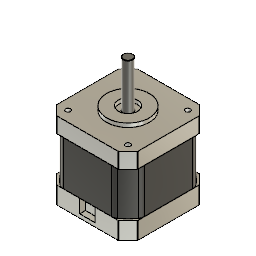
AquaMOCO-Slider-1-0-0 (Autodesk Fusion 360 archive; units mm, degrees)
design "Nema17_40mm_V2"
Autodesk Fusion 360 part; units mm, degrees
note: some values were not read from the file. Chosen so that the rebuilt part matches the saved one: how an offset face is resized.
sketch "Sketch1" plane through (0, 0, 0) normal (0, 0, 1) x (1, 0, 0) in component "Component"
  line L0 (16, 21) -> (-16, 21)
  line L1 (-21, 16) -> (-21, -16)
  line L2 (-16, -21) -> (16, -21)
  line L3 (21, -16) -> (21, 16)
  line L4 (21, 21) -> (-21, -21) construction
  line L5 (-21, 21) -> (21, -21) construction
  line L6 (-15.6506, 22.8547) -> (-16, 22.8547)
  line L7 (-21, 16) -> (-16, 21)
  line L8 (21, 16) -> (16, 21)
  line L9 (-16, -21) -> (-21, -16)
  line L10 (16, -21) -> (21, -16)
  circle A0 centre (-15.5, 15.5) radius 1.5
  circle A1 centre (15.5, 15.5) radius 1.5
  circle A2 centre (15.5, -15.5) radius 1.5
  circle A3 centre (-15.5, -15.5) radius 1.5
  circle A4 centre (0, 0) radius 11
  circle A5 centre (0, 0) radius 5
  circle A6 centre (0, 0) radius 2.5
  line L11 (-15.5, 15.5) -> (24, 15.5) construction
  line L12 (-15.5, -15.5) -> (24, -15.5) construction
  line L13 (15.5, 29) -> (15.5, -23) construction
  dimension "d3" = 3
  dimension "d4" = 15.5
  dimension "d5" = 15.5
  dimension "d6" = 5
  dimension "d58" = 15.5
  measures "d3" diameter of A0
  measures "d4" distance of A4.centre A0.centre
  measures "d5" distance of A4.centre A0.centre
  measures "d6" diameter of A6
  measures "d58" distance of A4.centre L13
extrude "Extrude1" add sketch "Sketch1" along normal blind 2 contours A4 makes body 1 in component "Component"
extrude "Extrude2" add sketch "Sketch1" along normal blind 24 separate body contours A6 makes body 2 in component "Component"
extrude "Extrude3" add sketch "Sketch1" against normal blind 1 separate body contours A5 makes body 3 in component "Component"
extrude "Extrude4" add sketch "Sketch1" against normal blind 8 contours L0 L1 L2 L3 L7 L8 L9 L10 | A4 bodies 1 3 in component "Component"
sketch "Sketch2" plane through (0, 0, -8) normal (0, 0, -1) x (1, 0, 0) in component "Component"
  circle A0 centre (15.5, 15.5) radius 1.5
  circle A1 centre (15.5, -15.5) radius 1.5
  circle A2 centre (0, 0) radius 5
  circle A3 centre (-15.5, 15.5) radius 1.5
  circle A4 centre (-15.5, -15.5) radius 1.5
  line L0 (16, 21) -> (-16, 21)
  line L1 (-16, 21) -> (-21, 16)
  line L2 (-21, 16) -> (-21, -16)
  line L3 (-21, -16) -> (-16, -21)
  line L4 (-16, -21) -> (16, -21)
  line L5 (16, -21) -> (21, -16)
  line L6 (21, -16) -> (21, 16)
  line L7 (21, 16) -> (16, 21)
  line L8 (12.4984, 21) -> (-12.4984, 21)
  line L9 (-21, 12.4984) -> (-21, -12.4984)
  line L10 (-12.4984, -21) -> (12.4984, -21)
  line L11 (21, -12.4984) -> (21, 12.4984)
  line L12 (21, 21) -> (-21, -21) construction
  line L13 (-21, 21) -> (21, -21) construction
  arc A5 (-14.8678, 20.2227) -> (-20.2227, 14.8678) centre (0, 0) ccw
  arc A6 (20.2227, 14.8678) -> (14.8678, 20.2227) centre (0, 0) ccw
  arc A7 (-20.2227, -14.8678) -> (-14.8678, -20.2227) centre (0, 0) ccw
  arc A8 (14.8678, -20.2227) -> (21, -13.7481) centre (0, 0) ccw
  arc A9 (-12.4984, 21) -> (-14.8678, 20.2227) centre (-12.4984, 17) ccw
  arc A10 (-20.2227, 14.8678) -> (-21, 12.4984) centre (-17, 12.4984) ccw
  arc A11 (14.8678, 20.2227) -> (12.4984, 21) centre (12.4984, 17) ccw
  arc A12 (20.2227, -14.8678) -> (21, -12.4984) centre (17, -12.4984) ccw
  arc A13 (21, 12.4984) -> (20.2227, 14.8678) centre (17, 12.4984) ccw
  arc A14 (12.4984, -21) -> (14.8678, -20.2227) centre (12.4984, -17) ccw
  arc A15 (-14.8678, -20.2227) -> (-12.4984, -21) centre (-12.4984, -17) ccw
  arc A16 (-21, -12.4984) -> (-20.2227, -14.8678) centre (-17, -12.4984) ccw
  dimension "d15" = 42
  dimension "d16" = 42
  dimension "d17" = 50.2
  dimension "d18" = 4
  dimension "d19" = 4
  dimension "d20" = 4
  dimension "d21" = 4
  dimension "d22" = 4
  dimension "d23" = 4
  dimension "d24" = 4
  dimension "d25" = 4
  measures "d15" distance of L12.end L13.end
  measures "d16" distance of L13.start L12.end
  measures "d17" diameter of A5
  measures "d18" radius of A9
  measures "d19" radius of A10
  measures "d20" radius of A11
  measures "d21" radius of A12
  measures "d22" radius of A13
  measures "d23" radius of A14
  measures "d24" radius of A15
  measures "d25" radius of A16
extrude "Extrude5" add sketch "Sketch2" along normal blind 23 separate body contours A0 | A1 | A2 | A3 | A4 | L0 L2 L4 L6 L8 L9 L10 L11 A5 A6 A7 A8 A9 A10 A11 A12 A13 A14 A15 A16 makes body 4 in component "Component"
ref_plane "WorkPlane1" through (0, 0, -40) normal (0, 0, 1) x (1, 0, 0) in component "Component"
sketch "Sketch3" plane through (-15.5, 15.5, -40) normal (0, 0, 1) x (1, 0, 0) in component "Component"
  circle A0 centre (15.5, -15.5) radius 4.75
  line L0 (31.5, -36.5) -> (-0.5, -36.5)
  line L1 (-0.5, -36.5) -> (-5.5, -31.5)
  line L2 (-5.5, -31.5) -> (-5.5, 0.5)
  line L3 (-5.5, 0.5) -> (-0.5, 5.5)
  line L4 (-0.5, 5.5) -> (31.5, 5.5)
  line L5 (31.5, 5.5) -> (36.5, 0.5)
  line L6 (36.5, 0.5) -> (36.5, -31.5)
  line L7 (36.5, -31.5) -> (31.5, -36.5)
  circle A1 centre (31, -31) radius 3
  circle A2 centre (31, 0) radius 3
  circle A3 centre (0, -31) radius 3
  circle A4 centre (0, 0) radius 3
  dimension "d29" = 6
  dimension "d30" = 6
  dimension "d31" = 6
  dimension "d32" = 6
  dimension "d33" = 9.5
  measures "d29" diameter of A1
  measures "d30" diameter of A2
  measures "d31" diameter of A3
  measures "d32" diameter of A4
  measures "d33" diameter of A0
extrude "Extrude6" add sketch "Sketch3" along normal blind 9 separate body contours A0 | L0 L1 L2 L3 L4 L5 L6 L7 | A1 | A2 | A3 | A4 makes body 5 in component "Component"
extrude "Extrude8" cut sketch "Sketch3" along normal blind 3 contours A1 | A2 | A3 | A4 bodies 5 in component "Component"
extrude "Extrude9" cut sketch "Sketch3" along normal blind 3.5 contours A0 bodies 5 in component "Component"
chamfer "Chamfer1" distance 0.2 angle 45 1 edges at (-2.3308, -0.904, 24) on bodies 2 in component "Component"
fillet "Fillet1" radius 0.5 16 edges at (16, 21, -4) (21, 16, -4) (21, -16, -4) (16, -21, -4) (-16, -21, -4) (-21, -16, -4) (-21, 16, -4) (-16, 21, -4) (16, 21, -35.5) (21, 16, -35.5) (21, -16, -35.5) (16, -21, -35.5) (-21, -16, -35.5) (-16, -21, -35.5) (-16, 21, -35.5) (-21, 16, -35.5) on bodies 1 5 in component "Component"
sketch "Sketch4" plane through (0, -21, 0) normal (0, -1, 0) x (1, 0, 0) in component "Component"
  line L0 (-15.7929, -31) -> (-15.7929, -40)
  line L1 (-15.7929, -40) -> (15.7929, -40)
  line L2 (15.7929, -40) -> (15.7929, -31)
  line L3 (15.7929, -31) -> (-15.7929, -31)
  line L4 (-4, -31) -> (4, -31)
  line L5 (4, -31) -> (4, -38)
  line L6 (4, -38) -> (-4, -38)
  line L7 (-4, -38) -> (-4, -31)
  line L8 (0, -40) -> (0, -26) construction
  dimension "d53" = 8
  dimension "d54" = 7
  dimension "d55" = 4
  measures "d53" distance of L4.start L4.end
  measures "d54" distance of L4.start L6.end
  measures "d55" distance of L5 L8
extrude "Extrude10" cut sketch "Sketch4" against normal blind 3 contours L3 L4 L5 L6 L7 bodies 5 in component "Component"
thread "Thread1" "ISO Metric profile 3.0 M3x0.5 6H" major diameter 3.086 minor diameter 2.529 pitch 0.5 angle 60 resizes the face on face at (-14.0019, -15.5748, -5.3333) on bodies 1 in component "Component"
thread "Thread2" "ISO Metric profile 3.0 M3x0.5 6H" major diameter 3.086 minor diameter 2.529 pitch 0.5 angle 60 resizes the face on face at (16.9981, -15.5748, -5.3333) on face at (16.9981, 15.4252, -5.3333) on face at (-14.0019, 15.4252, -5.3333) on bodies 1 in component "Component"
component "Component" placed x (1, 0, 0) y (0, 1, 0) z (0, 0, 1) at (0, 0, 0)
equation "d4 = ( 31 / 2 ) * 1 mm"
equation "d5 = d4"
equation "d9 = AxleLength"
equation "d13 = -FrontCoverLength"
equation "d26 = MotorLength - BackCoverLength - FrontCoverLength"
equation "d28 = -MotorLength"
equation "d34 = BackCoverLength"
equation "MotorLength = 40 mm"
equation "AxleLength = 24 mm" comment "Axle Length From Flange"
equation "FrontCoverLength = 8 mm"
equation "BackCoverLength = 9 mm"
